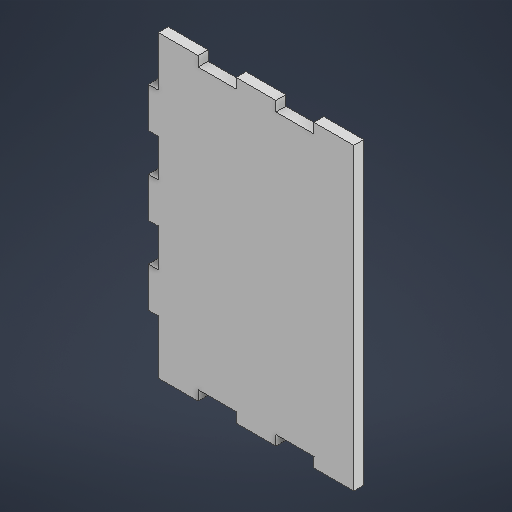
# Autodesk Inventor part: part4
Saved by Autodesk Inventor 2027.1 (Build 311270010, 270A)
## iProperties
Created: 2026-10-07
Part Number: part4
Material: Generic
Document SubType Name: Modeling
Designer: daniel
Density: 1 g/cm^3
Appearance: Default
Author: daniel
Autodesk Inventor part; units mm, degrees
ref_plane "YZ Plane" through (0, 0, 0) normal (1, 0, 0) x (0, 1, 0)
ref_plane "XZ Plane" through (0, 0, 0) normal (0, 1, 0) x (-1, 0, 0)
ref_plane "XY Plane" through (0, 0, 0) normal (0, 0, 1) x (1, 0, 0)
sketch "Sketch1" plane through (0, 0, 0) normal (0, 0, 1) x (1, 0, 0)
  line L0 (-50, 75) -> (50, 75)
  line L1 (50, 75) -> (50, -75)
  line L2 (50, -75) -> (-50, -75)
  line L3 (-50, -75) -> (-50, 75)
  line L4 (-50, 75) -> (-45, 75)
  line L5 (-45, 75) -> (-45, 50)
  line L6 (-45, 50) -> (-50, 50)
  line L7 (-50, 50) -> (-50, 75)
  line L8 (-50, 50) -> (-45, 50)
  line L9 (-45, 50) -> (-45, 30)
  line L10 (-45, 30) -> (-50, 30)
  line L11 (-50, 30) -> (-50, 50)
  line L12 (-45, 30) -> (-50, 30)
  line L13 (-50, 30) -> (-50, 11)
  line L14 (-50, 11) -> (-45, 11)
  line L15 (-45, 11) -> (-45, 30)
  line L16 (-50, 11) -> (-45, 11)
  line L17 (-45, 11) -> (-45, -9)
  line L18 (-45, -9) -> (-50, -9)
  line L19 (-50, -9) -> (-50, 11)
  line L20 (-50, -9) -> (-45, -9)
  line L21 (-45, -9) -> (-45, -28)
  line L22 (-45, -28) -> (-50, -28)
  line L23 (-50, -28) -> (-50, -9)
  line L24 (-45, -28) -> (-50, -28)
  line L25 (-50, -28) -> (-50, -48)
  line L26 (-50, -48) -> (-45, -48)
  line L27 (-45, -48) -> (-45, -28)
  line L28 (-50, -48) -> (-45, -48)
  line L29 (-45, -48) -> (-45, -67)
  line L30 (-50, -67) -> (-50, -48)
  line L31 (-45, -67) -> (-45, -75)
  line L32 (-45, -75) -> (-50, -75)
  line L33 (-50, -75) -> (-50, -67)
  line L34 (-45, 75) -> (-25, 75)
  line L35 (-25, 75) -> (-25, 70)
  line L36 (-25, 70) -> (-45, 70)
  line L37 (-45, 70) -> (-45, 75)
  line L38 (-25, 70) -> (-6, 70)
  line L39 (-6, 70) -> (-6, 75)
  line L40 (-6, 75) -> (-25, 75)
  line L41 (-25, 75) -> (-25, 70)
  line L42 (-6, 70) -> (14, 70)
  line L43 (14, 70) -> (14, 75)
  line L44 (14, 75) -> (-6, 75)
  line L45 (-6, 75) -> (-6, 70)
  line L46 (14, 70) -> (33, 70)
  line L47 (33, 70) -> (33, 75)
  line L48 (33, 75) -> (14, 75)
  line L49 (14, 75) -> (14, 70)
  line L50 (33, 70) -> (50, 70)
  line L51 (50, 70) -> (50, 75)
  line L52 (50, 75) -> (33, 75)
  line L53 (33, 75) -> (33, 70)
  line L54 (50, 75) -> (53, 75)
  line L55 (53, 75) -> (53, 70)
  line L56 (53, 70) -> (50, 70)
  line L57 (50, 70) -> (50, 75)
  line L58 (53, 70) -> (53, -75)
  line L59 (53, -75) -> (50, -75)
  line L60 (0, 0) -> (92.6837, 0)
  line L61 (92.6837, 0) -> (-105.3184, 0)
  line L62 (53, -75) -> (33, -75)
  line L63 (33, -75) -> (33, -70)
  line L64 (33, -70) -> (53, -70)
  line L65 (53, -70) -> (53, -75)
  line L66 (33, -70) -> (14, -70)
  line L67 (14, -70) -> (14, -75)
  line L68 (14, -75) -> (33, -75)
  line L69 (33, -75) -> (33, -70)
  line L70 (14, -75) -> (-6, -75)
  line L71 (-6, -75) -> (-6, -70)
  line L72 (-6, -70) -> (14, -70)
  line L73 (14, -70) -> (14, -75)
  line L74 (-6, -75) -> (-25, -75)
  line L75 (-25, -75) -> (-25, -70)
  line L76 (-25, -70) -> (-6, -70)
  line L77 (-6, -70) -> (-6, -75)
  line L78 (-25, -75) -> (-45, -75)
  line L79 (-45, -75) -> (-45, -70)
  line L80 (-45, -70) -> (-25, -70)
  line L81 (-25, -70) -> (-25, -75)
  dimension "d0" = 100
  dimension "d1" = 150
  dimension "d2" = 75
  dimension "d3" = 50
  dimension "d4" = 5
  dimension "d5" = 25
  dimension "d6" = 20
  dimension "d7" = 19
  dimension "d8" = 20
  dimension "d9" = 19
  dimension "d10" = 20
  dimension "d11" = 19
  dimension "d12" = 20
  dimension "d13" = 5
  dimension "d14" = 19
  dimension "d15" = 20
  dimension "d16" = 19
  dimension "d17" = 17
  dimension "d18" = 3
  dimension "d19" = 20
  dimension "d20" = 5
  dimension "d21" = 19
  dimension "d22" = 20
  dimension "d23" = 19
  constraints: 164 end point, 38 parallel, 20 horizontal, 19 perpendicular, 16 point on line, 1 collinear, 1 vertical
  measures "d0" distance of L1.end L2.end
  measures "d1" distance of L0.end L1.end
  measures "d2" distance from line of L60.start L0
  measures "d3" distance from line of L1 L60.start
  measures "d4" distance of L5.end L6.end
  measures "d5" distance of L4.end L5.end
  measures "d6" distance of L8.end L9.end
  measures "d7" distance of L13.end L12.end
  measures "d8" distance of L16.end L17.end
  measures "d9" distance of L20.end L21.end
  measures "d10" distance of L25.end L24.end
  measures "d11" distance of L28.end L29.end
  measures "d12" distance of L35.end L36.end
  measures "d13" distance of L34.end L35.end
  measures "d14" distance of L40.end L39.end
  measures "d15" distance of L44.end L43.end
  measures "d16" distance of L48.end L47.end
  measures "d17" distance of L46.end L50.end
  measures "d18" distance of L55.end L56.end
  measures "d19" distance of L63.end L64.end
  measures "d20" distance of L62.end L63.end
  measures "d21" distance of L68.end L67.end
  measures "d22" distance of L71.end L72.end
  measures "d23" distance of L75.end L76.end
extrude "Extrusion1" add sketch "Sketch1" along normal blind 5 contours L0 L35 L36 L5 | L6 L9 L10 L3 | L36 L38 L42 L46 L50 L1 L60 L61 L17 L15 L9 L5 | L0 L43 L42 L39 | L14 L17 L61 L3 | L61 L17 L18 L3 | L0 L1 L50 L47 | L61 L60 L1 L64 L66 L72 L76 L80 L31 L29 L27 L21 L17 | L54 L55 L56 L1 | L22 L27 L26 L3 | L56 L58 L60 L1 | L60 L58 L64 L1 | L64 L58 L59 L1 | L1 L2 L63 L64 | L31 L80 L75 L2 | L67 L2 L71 L72
body "Solid1"
